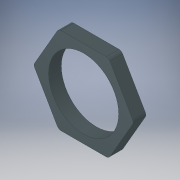
# Autodesk Inventor part: connector_nut
Saved by Autodesk Inventor 2017 (Build 210142000, 142)
## iProperties
Created: 2017-08-10
Part Number: connector_nut
Material: Lead
Document SubType Name: Modeling
Designer: Kai
Density: 11.34 g/cm^3
Appearance: Lead
Author: Kai
Autodesk Inventor part; units mm, degrees
ref_plane "YZ Plane" through (0, 0, 0) normal (1, 0, 0) x (0, 1, 0)
ref_plane "XZ Plane" through (0, 0, 0) normal (0, 1, 0) x (-1, 0, 0)
ref_plane "XY Plane" through (0, 0, 0) normal (0, 0, 1) x (1, 0, 0)
sketch "Sketch1" plane through (0, 0, 0) normal (0, 0, 1) x (1, 0, 0)
  circle A0 centre (0, 0) radius 10.5
  circle A1 centre (0, 0) radius 13 construction
  line L0 (7.8722, 12.365) -> (14.6445, 0.635)
  line L1 (14.6445, -0.635) -> (7.8722, -12.365)
  line L2 (6.7723, -13) -> (-6.7723, -13)
  line L3 (-7.8722, -12.365) -> (-14.6445, -0.635)
  line L4 (-14.6445, 0.635) -> (-7.8722, 12.365)
  line L5 (-6.7723, 13) -> (6.7723, 13)
  arc A2 (-6.7723, 13) -> (-7.8722, 12.365) centre (-6.7723, 11.73) ccw
  arc A3 (-14.6445, 0.635) -> (-14.6445, -0.635) centre (-13.5446, 0) ccw
  arc A4 (-7.8722, -12.365) -> (-6.7723, -13) centre (-6.7723, -11.73) ccw
  arc A5 (6.7723, -13) -> (7.8722, -12.365) centre (6.7723, -11.73) ccw
  arc A6 (14.6445, -0.635) -> (14.6445, 0.635) centre (13.5446, 0) ccw
  arc A7 (7.8722, 12.365) -> (6.7723, 13) centre (6.7723, 11.73) ccw
  point P0 (0, 13)
  point P1 (7.5056, 13)
  point P2 (15.0111, 0)
  point P3 (7.5056, -13)
  point P4 (-7.5056, -13)
  point P5 (-15.0111, 0)
  point P6 (-7.5056, 13)
  dimension "d1" = 26
  dimension "d0" = 21
  dimension "d2" = 1.27
  constraints: 12 end point, 12 point on circle, 12 point on line, 12 tangent, 7 centre point, 5 equal radius, 3 coincident, 1 midpoint, 1 vertical alignment, 15 other
  measures "d0" diameter of A0
  measures "d2" radius of A2
extrude "Extrusion1" add sketch "Sketch1" along normal blind 3.81
body "Solid1"
